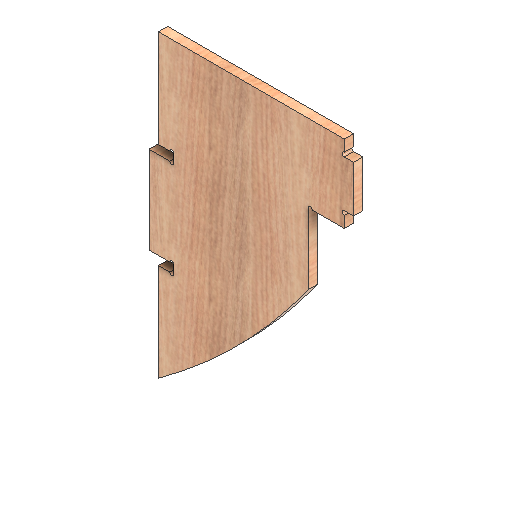
# Autodesk Inventor part: Support A1
Saved by Autodesk Inventor 2021 (Build 250183000, 183)
## iProperties
Created: 2020-05-09
Part Number: Support A1
Material: Wood (Birch)
Document SubType Name: Modeling
Designer: Dan Wikman
Density: 0.55 g/cm^3
Appearance: Birch - Natural Polished
Mass: 1430.75 g
Surface Area: 3239.05 cm^2
Volume: 2601.37 cm^3
Autodesk Inventor part; units mm, degrees
ref_plane "YZ Plane" through (0, 0, 0) normal (1, 0, 0) x (0, 1, 0)
ref_plane "XZ Plane" through (0, 0, 0) normal (0, 1, 0) x (-1, 0, 0)
ref_plane "XY Plane" through (0, 0, 0) normal (0, 0, 1) x (1, 0, 0)
sketch "CONTOURS" plane through (0, 0, 0) normal (0, 0, 1) x (1, 0, 0)
  arc A0 (354.6305, 1027.9401) -> (346.6305, 1027.9401) centre (350.6305, 1027.9401) ccw
  line L0 (346.6305, 1027.9401) -> (346.6305, 890.3591)
  arc A1 (56.6305, 596.8599) -> (346.6305, 890.3591) centre (-693.3695, 1627.9389) ccw
  line L1 (56.6305, 596.8599) -> (56.6305, 785.8598)
  line L2 (56.6305, 785.8598) -> (78.6305, 785.8598)
  arc A2 (78.6305, 785.8598) -> (86.6305, 785.8598) centre (82.6305, 785.8598) ccw
  line L3 (86.6305, 785.8598) -> (86.6305, 802.8598)
  arc A3 (86.6305, 802.8598) -> (78.6305, 802.8598) centre (82.6305, 802.8598) ccw
  line L4 (78.6305, 802.8598) -> (38.6305, 802.8598)
  line L5 (38.6305, 802.8598) -> (38.6305, 971.8598)
  line L6 (38.6305, 971.8598) -> (78.6305, 971.8598)
  arc A4 (78.6305, 971.8598) -> (86.6305, 971.8598) centre (82.6305, 971.8598) ccw
  line L7 (86.6305, 971.8598) -> (86.6305, 988.8598)
  arc A5 (86.6305, 988.8598) -> (78.6305, 988.8598) centre (82.6305, 988.8598) ccw
  line L8 (78.6305, 988.8598) -> (56.6305, 988.8598)
  line L9 (56.6305, 988.8598) -> (56.6305, 1177.8597)
  line L10 (56.6305, 1177.8597) -> (416.6305, 1177.8597)
  line L11 (416.6305, 1177.8597) -> (416.6305, 1155.9383)
  arc A6 (416.6305, 1155.9383) -> (416.6305, 1147.9383) centre (416.6305, 1151.9383) ccw
  line L12 (416.6305, 1147.9383) -> (434.6305, 1147.9383)
  line L13 (434.6305, 1147.9383) -> (434.6305, 1057.9383)
  line L14 (434.6305, 1057.9383) -> (416.6305, 1057.9383)
  arc A7 (416.6305, 1057.9383) -> (416.6305, 1049.9383) centre (416.6305, 1053.9383) ccw
  line L15 (416.6305, 1049.9383) -> (416.6305, 1027.9401)
  line L16 (416.6305, 1027.9401) -> (354.6305, 1027.9401)
  constraints: 34 end point, 16 point on circle, 8 centre point
sketch "LETTERS" plane through (0, 0, 0) normal (0, 0, 1) x (1, 0, 0)
  line L0 (214.8818, 1093.6309) -> (234.6305, 1102.9383)
  line L1 (234.6305, 1084.5494) -> (214.8818, 1093.6309)
  line L2 (214.8058, 1113.3691) -> (234.6305, 1113.3691)
  line L3 (217.3755, 1109.636) -> (214.8058, 1113.3691)
  line L4 (226.7124, 1099.1165) -> (226.7124, 1088.2213)
  constraints: 10 end point, 1 perpendicular
extrude "Extrusion1" add sketch "CONTOURS" along normal blind 18
body "Solid1"
